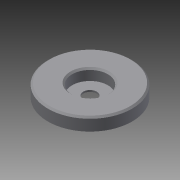
# Autodesk Inventor part: SpoolHandle-wheel1
Saved by Autodesk Inventor 2014 (Build 180170000, 170)
## iProperties
Created: 2014-04-04
Part Number: SpoolHandle-wheel1
Material: Generic
Document SubType Name: Modeling
Designer: Krzysiek
Density: 1 g/cm^3
Appearance: Default
Author: Krzysiek
Autodesk Inventor part; units mm, degrees
ref_plane "YZ Plane" through (0, 0, 0) normal (1, 0, 0) x (0, 1, 0)
ref_plane "XZ Plane" through (0, 0, 0) normal (0, 1, 0) x (-1, 0, 0)
ref_plane "XY Plane" through (0, 0, 0) normal (0, 0, 1) x (1, 0, 0)
sketch "Sketch1" plane through (0, 0, 0) normal (0, 0, 1) x (1, 0, 0)
  circle A0 centre (0, 0) radius 26.5
  dimension "d0" = 53
  constraints: 1 centre point, 1 coincident
  measures "d0" diameter of A0
extrude "Extrusion1" add sketch "Sketch1" along normal blind 8
sketch "Sketch2" plane through (0, 0, 8) normal (0, 0, 1) x (1, 0, 0)
  circle A0 centre (0, 0) radius 26.5 projected
  circle A1 centre (0, 0) radius 4.25
  dimension "d3" = 8.5
  constraints: 1 centre point, 1 coincident
  measures "d3" diameter of A1
extrude "Extrusion2" cut sketch "Sketch2" against normal blind 8 contours A1
sketch "Sketch3" plane through (0, 0, 8) normal (0, 0, 1) x (1, 0, 0)
  circle A0 centre (0, 0) radius 4.25 projected
  circle A1 centre (0, 0) radius 26.5 projected
  circle A2 centre (0, 0) radius 11.25
  dimension "d6" = 22.5
  constraints: 1 centre point, 1 coincident
  measures "d6" diameter of A2
extrude "Extrusion3" cut sketch "Sketch3" against normal blind 7 contours A2
chamfer "Chamfer1" distance 1 angle 45 1 edges at (-11.25, 0, 8)
chamfer "Chamfer2" distance 1 angle 45 1 edges at (-26.5, 0, 8)
body "Solid1"
